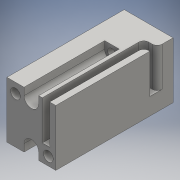
# Autodesk Inventor part: fourche_jonction_bas_haut
Saved by Autodesk Inventor 2016 (Build 200138000, 138)
## iProperties
Created: 2017-07-25
Part Number: fourche_jonction_bas_haut
Material: Generic
Document SubType Name: Modeling
Designer: mbouhier
Density: 1 g/cm^3
Appearance: Default
Author: mbouhier
Autodesk Inventor part; units mm, degrees
sketch "Sketch1" plane through (0, 0, 0) normal (0, 1, 0) x (-1, 0, 0)
  line L0 (-10, 11.5) -> (10, 11.5)
  line L1 (10, 11.5) -> (10, -11.5)
  line L2 (10, -11.5) -> (-10, -11.5)
  line L3 (-10, -11.5) -> (-10, 11.5)
  line L4 (-10, 11.5) -> (10, -11.5) construction
  line L5 (10, 11.5) -> (-10, -11.5) construction
  line L6 (-2.3726, 4.5) -> (2.3726, 4.5)
  line L7 (2.3726, 4.5) -> (2.3726, -4.5)
  line L8 (2.3726, -4.5) -> (-2.3726, -4.5)
  line L9 (-2.3726, -4.5) -> (-2.3726, 4.5)
  line L10 (-2.3726, 4.5) -> (2.3726, -4.5) construction
  line L11 (2.3726, 4.5) -> (-2.3726, -4.5) construction
  point P0 (0, 0)
  point P1 (6.5, 7.475)
  point P2 (-6.9565, -8)
  dimension "d19" = 4
  dimension "d0" = 20
  dimension "d1" = 23
  dimension "d2" = 9
  dimension "d4" = 3.5
  dimension "d41" = 3.5
  constraints: 24 end point, 4 midpoint, 4 parallel, 2 horizontal, 2 perpendicular, 2 point on line
  measures "d0" distance of L1.end L2.end
  measures "d1" distance of L0.end L1.end
  measures "d2" distance of L6.end L7.end
  measures "d4" distance from line of L2 point (-6.957, -8)
  measures "d41" distance from line of L1 point (6.5, 7.475)
extrude "Extrusion1" add sketch "Sketch1" along normal blind 48 contours L0 L1 L2 L3 | L6 L7 L8 L9
hole "Hole1" at (-6.5, 0, 7.475) at (6.9565, 0, -8) direction (0, 1, 0) diameter 4 depth 6 tip angle 118
ref_plane "Work Plane1" through (10.5, 0, 11.5) normal (1, 0, 0) x (0, 0, -1)
sketch "Sketch5" plane through (10.5, 0, 11.5) normal (1, 0, 0) x (0, 0, -1)
  line L0 (6.5, 38) -> (15.5, 38)
  line L1 (15.5, 38) -> (15.5, 42)
  line L2 (15.5, 42) -> (6.5, 42)
  line L3 (6.5, 42) -> (6.5, 38)
  line L4 (6.5, 38) -> (15.5, 42) construction
  line L5 (15.5, 38) -> (6.5, 42) construction
  line L6 (0, 48) -> (23, 48) projected
  point P0 (11.5, 0)
  point P1 (11, 40)
  dimension "d18" = 9
  dimension "d19" = 4
  dimension "d20" = 8
  constraints: 12 end point, 2 midpoint, 2 parallel, 1 horizontal, 1 perpendicular
  measures "d18" distance of L2.end L1.end
  measures "d19" distance of L1.end L0.end
  measures "d20" distance from line of point (11, 40) L6
ref_plane "Work Plane2" through (-10, 0, 0) normal (0, 0, 1) x (1, 0, 0)
sketch "Sketch7" plane through (0, 48, 0) normal (0, 1, 0) x (1, 0, 0)
  point P0 (0, 0)
sketch "Sketch8" plane through (0, 48, 0) normal (0, 1, 0) x (1, 0, 0)
  line L0 (-10, -11.5) -> (10, -11.5) projected
  line L1 (10, 11.5) -> (-10, 11.5) projected
  line L2 (-2.3726, 48) -> (9.101, 48) projected
  line L3 (-2.3726, 48) -> (9.101, 48) projected
  line L4 (9.101, 4.5) -> (9.101, -4.5) projected
  point P0 (0, 0)
  point P1 (0, 8.5)
  point P2 (0, -8.5)
  point P3 (2.3726, -4.5)
  point P4 (2.3726, 4.5)
  point P5 (-2.3726, -4.5)
  point P6 (-2.3726, 4.5)
  dimension "d30" = 3
  dimension "d31" = 3
  constraints: 1 vertical alignment, 2 other
  measures "d30" distance from line of L1 point (0, 8.5)
  measures "d31" distance from line of L0 point (0, -8.5)
ref_plane "Work Plane3" through (0, 33, 0) normal (0, 1, 0) x (1, 0, 0)
hole "Hole2" at (0, 48, -8.5) at (0, 48, 8.5) direction (0, -1, 0) diameter 3.5 depth 15
sketch "Sketch9" plane through (0, 33, 0) normal (0, 1, 0) x (1, 0, 0)
  circle A0 centre (0, 8.5) radius 1.75 projected
  circle A1 centre (0, -8.5) radius 1.75 projected
  circle A2 centre (0, -8.5) radius 1.75 projected
  circle A3 centre (0, -8.5) radius 3
  circle A4 centre (0, 8.5) radius 3
  line L0 (-3, 8.5) -> (3, 8.5)
  line L1 (3, 8.5) -> (3, 11.5)
  line L2 (3, 11.5) -> (-3, 11.5)
  line L3 (-3, 11.5) -> (-3, 8.5)
  line L4 (10, -11.5) -> (-10, -11.5) projected
  line L5 (-3, -8.5) -> (3, -8.5)
  line L6 (3, -8.5) -> (3, -11.5)
  line L7 (3, -11.5) -> (-3, -11.5)
  line L8 (-3, -11.5) -> (-3, -8.5)
  point P0 (0, 0)
  constraints: 16 end point, 4 parallel, 3 point on line, 2 coincident, 2 horizontal, 2 horizontal alignment, 2 perpendicular, 4 other
extrude "Extrusion3" cut sketch "Sketch9" against normal blind 25
sketch "Sketch11" plane through (-10, 0, 11.5) normal (0, 0, 1) x (1, 0, 0)
  line L0 (7, 33) -> (13, 33) projected
  line L1 (13, 33) -> (13, 8) projected
  line L2 (13, 8) -> (7, 8) projected
  line L3 (7, 8) -> (7, 33) projected
  line L4 (20, 0) -> (0, 0) projected
  line L5 (20, 0) -> (20, 48) projected
  line L6 (0, 48) -> (20, 48) projected
  line L7 (0, 0) -> (0, 48) projected
  line L8 (20, 0) -> (20, 48) projected
  line L9 (20, 0) -> (0, 0) projected
  line L10 (14.9565, 0) -> (14.9565, 6) projected
  line L11 (14.5, 6) -> (14.5, 41.5)
  line L12 (14.5, 41.5) -> (20, 41.5)
  line L13 (17.5, 3) -> (17.5, 38.5)
  line L14 (17.5, 38.5) -> (20, 38.5)
  line L15 (17.5, 3) -> (17.5, 0)
  line L16 (14.5, 0) -> (17.5, 0)
  line L17 (14.5, 0) -> (14.5, 6)
  point P0 (10, 0)
  point P1 (20, 40)
  dimension "d42" = 8
  dimension "d43" = 1.5
  dimension "d44" = 1.5
  dimension "d48" = 3
  dimension "d49" = 2.5
  constraints: 14 end point, 5 point on line, 4 perpendicular, 1 collinear, 1 vertical
  measures "d42" distance from line of point (20, 40) L6
  measures "d43" distance of point (20, 40) L12.end
  measures "d44" distance of point (20, 40) L14.end
  measures "d48" distance from line of L13.start L11
  measures "d49" distance between parallel lines of L13 L5
ref_plane "Work Plane4" through (-10, 0, -4.5) normal (0, 0, 1) x (1, 0, 0)
extrude "Extrusion4" cut sketch "Sketch11" against normal up to surface (16 mm away) contours L4 L17 L11 L12 L5 L14 L13 L15
fillet "Fillet1" radius 2 3 edges at (4.5, 41.5, 3.5) (10, 41.5, 3.5) (7.5, 38.5, 3.5)
sketch "Sketch12" plane through (0, 8, 0) normal (0, 1, 0) x (1, 0, 0)
  line L0 (3, -8.5) -> (3, -11.5) projected
  arc A0 (3, -8.5) -> (-3, -8.5) centre (0, -8.5) ccw projected
  line L1 (-3, -11.5) -> (-3, -8.5) projected
  line L2 (3, -11.5) -> (-3, -11.5) projected
  line L3 (-3, 8.5) -> (-3, 11.5) projected
  arc A1 (-3, 8.5) -> (3, 8.5) centre (0, 8.5) ccw projected
  line L4 (3, 11.5) -> (3, 8.5) projected
  line L5 (-3, 11.5) -> (3, 11.5) projected
  point P0 (0, 0)
extrude "Extrusion5" cut sketch "Sketch12" against normal blind 15
equation "\"d4\" = d3"
equation "\"d44\" = d43"
equation "\"d48\" = d47"
equation "\"d47\" = 2 * d45"
equation "\"d45\" = 1.5"
equation "\"d3\" = 3.5"
body "Solid1"
